Autodesk Inventor part; units mm, degrees
(part 3 of 6)
  spline S90 degree 5 poles (158.3441, 85.8402) (158.3513, 85.8419) (158.4053, 85.8546) (158.5062, 85.8783) (158.6539, 85.9125) (158.8488, 85.9569) (159.0837, 86.0091) (159.319, 86.0602) (159.5547, 86.1103) (159.7908, 86.1593) (160.0273, 86.2072) (160.2642, 86.2541) (160.5015, 86.3) (160.7391, 86.3449) (160.9771, 86.3887) (161.2155, 86.4315) (161.4542, 86.4734) (161.6932, 86.5143) (161.9326, 86.5542) (162.1723, 86.5932) (162.4124, 86.6312) (162.6527, 86.6682) (162.8934, 86.7044) (163.1343, 86.7396) (163.3756, 86.7739) (163.6172, 86.8073) (163.859, 86.8398) (164.1012, 86.8714) (164.3436, 86.9022) (164.5863, 86.932) (164.8293, 86.961) (165.0725, 86.9891) (165.3161, 87.0163) (165.5598, 87.0427) (165.8039, 87.0682) (166.0482, 87.0929) (166.2927, 87.1168) (166.5375, 87.1398) (166.7825, 87.162) (167.0278, 87.1834) (167.2733, 87.2039) (167.519, 87.2237) (167.765, 87.2426) (168.0604, 87.2644) (168.3069, 87.2815) (168.5042, 87.2946) (168.6523, 87.304) (168.7511, 87.3102) knots 0.383497 0.383497 0.383497 0.383497 0.383497 0.383497 0.385714 0.4 0.414286 0.428571 0.442857 0.457143 0.471429 0.485714 0.5 0.514286 0.528571 0.542857 0.557143 0.571429 0.585714 0.6 0.614286 0.628571 0.642857 0.657143 0.671429 0.685714 0.7 0.714286 0.728571 0.742857 0.757143 0.771429 0.785714 0.8 0.814286 0.828571 0.842857 0.857143 0.871429 0.885714 0.9 0.914286 0.928571 0.942857 0.957143 0.971429 1 1 1 1 1 1
  spline S91 degree 3 poles (156.5898, 86.6167) (156.7797, 86.2734) (157.3439, 85.8048) (158.0577, 85.7725) (158.3441, 85.8402) knots 0 0 0 0 0.571429 1 1 1 1
  arc A46 (156.5898, 86.6167) -> (155.8578, 87.927) centre (0, 0) ccw
  spline S92 degree 3 poles (156.1164, 89.828) (155.9086, 89.6196) (155.5618, 88.9948) (155.665, 88.2687) (155.8578, 87.927) knots 0 0 0 0 0.428571 1 1 1 1
  spline S93 degree 5 poles (156.1164, 89.828) (156.1216, 89.8333) (156.1608, 89.8726) (156.2338, 89.946) (156.3404, 90.0539) (156.4803, 90.1965) (156.648, 90.3692) (156.8149, 90.5427) (156.9811, 90.7172) (157.1466, 90.8926) (157.3115, 91.0689) (157.4756, 91.246) (157.6391, 91.424) (157.8019, 91.6028) (157.964, 91.7825) (158.1254, 91.963) (158.2862, 92.1443) (158.4464, 92.3264) (158.6059, 92.5094) (158.7647, 92.693) (158.923, 92.8775) (159.0805, 93.0627) (159.2375, 93.2487) (159.3938, 93.4354) (159.5495, 93.6229) (159.7046, 93.8111) (159.8591, 94) (160.013, 94.1896) (160.1663, 94.3799) (160.3189, 94.571) (160.471, 94.7627) (160.6225, 94.9551) (160.7733, 95.1482) (160.9236, 95.3419) (161.0733, 95.5363) (161.2224, 95.7314) (161.371, 95.9271) (161.5189, 96.1235) (161.6663, 96.3205) (161.8131, 96.5181) (161.9593, 96.7164) (162.1049, 96.9153) (162.25, 97.1148) (162.4234, 97.355) (162.5673, 97.5559) (162.6819, 97.7171) (162.7676, 97.8382) (162.8246, 97.9191) knots 0.383497 0.383497 0.383497 0.383497 0.383497 0.383497 0.385714 0.4 0.414286 0.428571 0.442857 0.457143 0.471429 0.485714 0.5 0.514286 0.528571 0.542857 0.557143 0.571429 0.585714 0.6 0.614286 0.628571 0.642857 0.657143 0.671429 0.685714 0.7 0.714286 0.728571 0.742857 0.757143 0.771429 0.785714 0.8 0.814286 0.828571 0.842857 0.857143 0.871429 0.885714 0.9 0.914286 0.928571 0.942857 0.957143 0.971429 1 1 1 1 1 1
  arc A47 (162.8246, 97.9191) -> (160.7388, 101.3067) centre (0, 0) ccw
  spline S94 degree 5 poles (150.4939, 98.9594) (150.501, 98.9618) (150.5537, 98.9791) (150.6522, 99.0112) (150.7965, 99.0578) (150.9869, 99.1185) (151.2165, 99.1905) (151.4466, 99.2614) (151.6772, 99.3313) (151.9084, 99.4001) (152.14, 99.4679) (152.372, 99.5348) (152.6045, 99.6006) (152.8375, 99.6654) (153.0709, 99.7293) (153.3048, 99.7922) (153.5391, 99.8541) (153.7738, 99.9152) (154.009, 99.9752) (154.2445, 100.0344) (154.4804, 100.0926) (154.7168, 100.1499) (154.9535, 100.2064) (155.1906, 100.2619) (155.4281, 100.3165) (155.666, 100.3703) (155.9042, 100.4232) (156.1428, 100.4752) (156.3817, 100.5264) (156.621, 100.5767) (156.8607, 100.6262) (157.1007, 100.6748) (157.341, 100.7226) (157.5817, 100.7696) (157.8227, 100.8157) (158.064, 100.861) (158.3056, 100.9056) (158.5476, 100.9492) (158.7898, 100.9921) (159.0324, 101.0342) (159.2753, 101.0755) (159.5184, 101.1161) (159.7619, 101.1558) (160.0544, 101.2025) (160.2985, 101.2405) (160.4941, 101.2703) (160.6409, 101.2922) (160.7388, 101.3067) knots 0.383497 0.383497 0.383497 0.383497 0.383497 0.383497 0.385714 0.4 0.414286 0.428571 0.442857 0.457143 0.471429 0.485714 0.5 0.514286 0.528571 0.542857 0.557143 0.571429 0.585714 0.6 0.614286 0.628571 0.642857 0.657143 0.671429 0.685714 0.7 0.714286 0.728571 0.742857 0.757143 0.771429 0.785714 0.8 0.814286 0.828571 0.842857 0.857143 0.871429 0.885714 0.9 0.914286 0.928571 0.942857 0.957143 0.971429 1 1 1 1 1 1
  spline S95 degree 3 poles (148.6801, 99.5844) (148.8984, 99.2584) (149.5003, 98.8394) (150.2143, 98.8677) (150.4939, 98.9594) knots 0 0 0 0 0.571429 1 1 1 1
  arc A48 (148.6801, 99.5844) -> (147.8396, 100.8279) centre (0, 0) ccw
  spline S96 degree 3 poles (147.936, 102.744) (147.7466, 102.5187) (147.4541, 101.8668) (147.6185, 101.1521) (147.8396, 100.8279) knots 0 0 0 0 0.428571 1 1 1 1
  spline S97 degree 5 poles (147.936, 102.744) (147.9408, 102.7497) (147.9765, 102.7921) (148.043, 102.8715) (148.1401, 102.988) (148.2674, 103.1421) (148.4198, 103.3283) (148.5714, 103.5154) (148.7222, 103.7033) (148.8723, 103.8921) (149.0216, 104.0817) (149.1701, 104.2721) (149.3179, 104.4634) (149.4649, 104.6554) (149.6112, 104.8481) (149.7568, 105.0417) (149.9016, 105.236) (150.0457, 105.431) (150.1892, 105.6268) (150.3319, 105.8233) (150.4739, 106.0205) (150.6152, 106.2184) (150.7558, 106.4171) (150.8957, 106.6164) (151.035, 106.8164) (151.1736, 107.017) (151.3115, 107.2184) (151.4487, 107.4203) (151.5853, 107.623) (151.7212, 107.8263) (151.8565, 108.0302) (151.9911, 108.2347) (152.125, 108.4399) (152.2583, 108.6457) (152.391, 108.8521) (152.523, 109.0591) (152.6544, 109.2668) (152.7852, 109.475) (152.9153, 109.6838) (153.0448, 109.8931) (153.1737, 110.1031) (153.302, 110.3136) (153.4296, 110.5247) (153.582, 110.7787) (153.7083, 110.9911) (153.8088, 111.1614) (153.8839, 111.2894) (153.9339, 111.3749) knots 0.383497 0.383497 0.383497 0.383497 0.383497 0.383497 0.385714 0.4 0.414286 0.428571 0.442857 0.457143 0.471429 0.485714 0.5 0.514286 0.528571 0.542857 0.557143 0.571429 0.585714 0.6 0.614286 0.628571 0.642857 0.657143 0.671429 0.685714 0.7 0.714286 0.728571 0.742857 0.757143 0.771429 0.785714 0.8 0.814286 0.828571 0.842857 0.857143 0.871429 0.885714 0.9 0.914286 0.928571 0.942857 0.957143 0.971429 1 1 1 1 1 1
  arc A49 (153.9339, 111.3749) -> (151.5683, 114.5734) centre (0, 0) ccw
  spline S98 degree 5 poles (141.5594, 111.3657) (141.5662, 111.3686) (141.6173, 111.3903) (141.7127, 111.4307) (141.8525, 111.4894) (142.0371, 111.566) (142.2598, 111.6572) (142.4831, 111.7474) (142.7069, 111.8366) (142.9314, 111.9248) (143.1564, 112.012) (143.382, 112.0982) (143.6081, 112.1835) (143.8347, 112.2679) (144.0619, 112.3513) (144.2896, 112.4339) (144.5178, 112.5154) (144.7465, 112.5961) (144.9756, 112.6759) (145.2053, 112.7549) (145.4355, 112.8329) (145.6661, 112.91) (145.8972, 112.9863) (146.1287, 113.0618) (146.3607, 113.1364) (146.5932, 113.2101) (146.8261, 113.283) (147.0594, 113.3551) (147.2931, 113.4263) (147.5273, 113.4968) (147.7619, 113.5664) (147.9969, 113.6352) (148.2323, 113.7032) (148.4681, 113.7704) (148.7043, 113.8368) (148.9409, 113.9025) (149.1779, 113.9673) (149.4153, 114.0314) (149.6531, 114.0946) (149.8912, 114.1572) (150.1297, 114.2189) (150.3685, 114.2799) (150.6078, 114.3401) (150.8953, 114.4115) (151.1353, 114.47) (151.3276, 114.5163) (151.472, 114.5506) (151.5683, 114.5734) knots 0.383497 0.383497 0.383497 0.383497 0.383497 0.383497 0.385714 0.4 0.414286 0.428571 0.442857 0.457143 0.471429 0.485714 0.5 0.514286 0.528571 0.542857 0.557143 0.571429 0.585714 0.6 0.614286 0.628571 0.642857 0.657143 0.671429 0.685714 0.7 0.714286 0.728571 0.742857 0.757143 0.771429 0.785714 0.8 0.814286 0.828571 0.842857 0.857143 0.871429 0.885714 0.9 0.914286 0.928571 0.942857 0.957143 0.971429 1 1 1 1 1 1
  spline S99 degree 3 poles (139.6991, 111.8346) (139.9443, 111.5283) (140.5796, 111.1618) (141.2886, 111.2506) (141.5594, 111.3657) knots 0 0 0 0 0.571429 1 1 1 1
  arc A50 (139.6991, 111.8346) -> (138.7562, 113.0023) centre (0, 0) ccw
  spline S100 degree 3 poles (138.6898, 114.9197) (138.5202, 114.6792) (138.284, 114.0048) (138.5084, 113.3066) (138.7562, 113.0023) knots 0 0 0 0 0.428571 1 1 1 1
  spline S101 degree 5 poles (138.6898, 114.9197) (138.6941, 114.9258) (138.726, 114.9711) (138.7856, 115.0558) (138.8724, 115.1802) (138.9862, 115.3445) (139.1223, 115.5429) (139.2575, 115.7422) (139.3918, 115.9423) (139.5253, 116.1431) (139.658, 116.3447) (139.7898, 116.547) (139.9209, 116.7501) (140.0511, 116.9538) (140.1805, 117.1583) (140.3091, 117.3635) (140.437, 117.5694) (140.564, 117.776) (140.6903, 117.9832) (140.8158, 118.1911) (140.9406, 118.3997) (141.0646, 118.6088) (141.1879, 118.8187) (141.3104, 119.0291) (141.4322, 119.2402) (141.5533, 119.4519) (141.6736, 119.6642) (141.7932, 119.8771) (141.9121, 120.0906) (142.0303, 120.3047) (142.1478, 120.5193) (142.2646, 120.7346) (142.3806, 120.9504) (142.496, 121.1667) (142.6107, 121.3836) (142.7247, 121.6011) (142.838, 121.8191) (142.9507, 122.0377) (143.0626, 122.2568) (143.1739, 122.4764) (143.2845, 122.6965) (143.3944, 122.9171) (143.5037, 123.1383) (143.6341, 123.4043) (143.7419, 123.6266) (143.8276, 123.8049) (143.8916, 123.9388) (143.9341, 124.0281) knots 0.383497 0.383497 0.383497 0.383497 0.383497 0.383497 0.385714 0.4 0.414286 0.428571 0.442857 0.457143 0.471429 0.485714 0.5 0.514286 0.528571 0.542857 0.557143 0.571429 0.585714 0.6 0.614286 0.628571 0.642857 0.657143 0.671429 0.685714 0.7 0.714286 0.728571 0.742857 0.757143 0.771429 0.785714 0.8 0.814286 0.828571 0.842857 0.857143 0.871429 0.885714 0.9 0.914286 0.928571 0.942857 0.957143 0.971429 1 1 1 1 1 1
  arc A51 (143.9341, 124.0281) -> (141.3058, 127.0145) centre (0, 0) ccw
  spline S102 degree 5 poles (131.6049, 122.9696) (131.6115, 122.9731) (131.6606, 122.999) (131.7522, 123.0473) (131.8865, 123.1177) (132.0639, 123.2097) (132.2781, 123.3194) (132.4929, 123.4282) (132.7084, 123.5361) (132.9246, 123.643) (133.1414, 123.749) (133.3588, 123.854) (133.5769, 123.9582) (133.7956, 124.0615) (134.0148, 124.1639) (134.2347, 124.2654) (134.4552, 124.3661) (134.6762, 124.4659) (134.8978, 124.5648) (135.1199, 124.6629) (135.3426, 124.7602) (135.5659, 124.8566) (135.7897, 124.9523) (136.014, 125.0471) (136.2388, 125.1411) (136.4642, 125.2342) (136.6901, 125.3266) (136.9164, 125.4182) (137.1433, 125.5091) (137.3706, 125.5991) (137.5985, 125.6884) (137.8268, 125.7768) (138.0556, 125.8646) (138.2849, 125.9515) (138.5146, 126.0377) (138.7448, 126.1232) (138.9754, 126.2079) (139.2065, 126.2919) (139.438, 126.3751) (139.67, 126.4576) (139.9024, 126.5393) (140.1352, 126.6203) (140.3685, 126.7006) (140.6489, 126.7961) (140.8831, 126.8748) (141.0708, 126.9372) (141.2117, 126.9837) (141.3058, 127.0145) knots 0.383497 0.383497 0.383497 0.383497 0.383497 0.383497 0.385714 0.4 0.414286 0.428571 0.442857 0.457143 0.471429 0.485714 0.5 0.514286 0.528571 0.542857 0.557143 0.571429 0.585714 0.6 0.614286 0.628571 0.642857 0.657143 0.671429 0.685714 0.7 0.714286 0.728571 0.742857 0.757143 0.771429 0.785714 0.8 0.814286 0.828571 0.842857 0.857143 0.871429 0.885714 0.9 0.914286 0.928571 0.942857 0.957143 0.971429 1 1 1 1 1 1
  spline S103 degree 3 poles (129.7116, 123.279) (129.9819, 122.9946) (130.646, 122.6833) (131.3448, 122.8319) (131.6049, 122.9696) knots 0 0 0 0 0.571429 1 1 1 1
  arc A52 (129.7116, 123.279) -> (128.6731, 124.3626) centre (0, 0) ccw
  spline S104 degree 3 poles (128.4443, 126.2674) (128.2957, 126.0134) (128.1176, 125.3214) (128.4004, 124.6447) (128.6731, 124.3626) knots 0 0 0 0 0.428571 1 1 1 1
  spline S105 degree 5 poles (128.4443, 126.2674) (128.448, 126.2738) (128.476, 126.3217) (128.5282, 126.4112) (128.6042, 126.5424) (128.7036, 126.7158) (128.8224, 126.9251) (128.9402, 127.1351) (129.0571, 127.3458) (129.173, 127.5573) (129.2881, 127.7694) (129.4024, 127.9821) (129.5157, 128.1956) (129.6282, 128.4097) (129.7398, 128.6244) (129.8505, 128.8398) (129.9605, 129.0558) (130.0695, 129.2724) (130.1778, 129.4895) (130.2852, 129.7073) (130.3919, 129.9257) (130.4977, 130.1447) (130.6027, 130.3642) (130.707, 130.5843) (130.8104, 130.8049) (130.9131, 131.0261) (131.015, 131.2479) (131.1161, 131.4702) (131.2165, 131.693) (131.3161, 131.9163) (131.415, 132.1401) (131.5131, 132.3645) (131.6104, 132.5894) (131.707, 132.8147) (131.8029, 133.0406) (131.898, 133.2669) (131.9925, 133.4938) (132.0862, 133.7211) (132.1791, 133.9489) (132.2714, 134.1771) (132.3629, 134.4059) (132.4538, 134.635) (132.5439, 134.8647) (132.6512, 135.1408) (132.7398, 135.3714) (132.81, 135.5563) (132.8624, 135.6951) (132.8972, 135.7878) knots 0.383497 0.383497 0.383497 0.383497 0.383497 0.383497 0.385714 0.4 0.414286 0.428571 0.442857 0.457143 0.471429 0.485714 0.5 0.514286 0.528571 0.542857 0.557143 0.571429 0.585714 0.6 0.614286 0.628571 0.642857 0.657143 0.671429 0.685714 0.7 0.714286 0.728571 0.742857 0.757143 0.771429 0.785714 0.8 0.814286 0.828571 0.842857 0.857143 0.871429 0.885714 0.9 0.914286 0.928571 0.942857 0.957143 0.971429 1 1 1 1 1 1
  arc A53 (132.8972, 135.7878) -> (130.0251, 138.5405) centre (0, 0) ccw
  spline S106 degree 5 poles (120.7023, 133.6875) (120.7086, 133.6915) (120.7552, 133.7215) (120.8424, 133.7774) (120.9703, 133.8589) (121.1393, 133.9656) (121.3433, 134.0931) (121.5482, 134.2197) (121.7538, 134.3455) (121.9601, 134.4703) (122.1671, 134.5943) (122.3748, 134.7175) (122.5833, 134.8398) (122.7924, 134.9612) (123.0022, 135.0818) (123.2127, 135.2016) (123.4238, 135.3206) (123.6356, 135.4388) (123.848, 135.5562) (124.061, 135.6728) (124.2747, 135.7886) (124.4889, 135.9036) (124.7038, 136.0179) (124.9193, 136.1314) (125.1353, 136.2441) (125.352, 136.3561) (125.5692, 136.4673) (125.787, 136.5777) (126.0053, 136.6875) (126.2242, 136.7965) (126.4437, 136.9047) (126.6637, 137.0123) (126.8842, 137.1191) (127.1053, 137.2252) (127.3268, 137.3305) (127.5489, 137.4352) (127.7716, 137.5392) (127.9947, 137.6424) (128.2183, 137.745) (128.4425, 137.8468) (128.6671, 137.948) (128.8922, 138.0485) (129.1178, 138.1483) (129.3891, 138.2672) (129.6158, 138.3655) (129.7975, 138.4435) (129.934, 138.5018) (130.0251, 138.5405) knots 0.383497 0.383497 0.383497 0.383497 0.383497 0.383497 0.385714 0.4 0.414286 0.428571 0.442857 0.457143 0.471429 0.485714 0.5 0.514286 0.528571 0.542857 0.557143 0.571429 0.585714 0.6 0.614286 0.628571 0.642857 0.657143 0.671429 0.685714 0.7 0.714286 0.728571 0.742857 0.757143 0.771429 0.785714 0.8 0.814286 0.828571 0.842857 0.857143 0.871429 0.885714 0.9 0.914286 0.928571 0.942857 0.957143 0.971429 1 1 1 1 1 1
  spline S107 degree 3 poles (118.7895, 133.8352) (119.083, 133.5748) (119.771, 133.3209) (120.4548, 133.5282) (120.7023, 133.6875) knots 0 0 0 0 0.571429 1 1 1 1
  arc A54 (118.7895, 133.8352) -> (117.6628, 134.8268) centre (0, 0) ccw
  spline S108 degree 3 poles (117.2733, 136.7053) (117.1468, 136.4396) (117.028, 135.7351) (117.3672, 135.0848) (117.6628, 134.8268) knots 0 0 0 0 0.428571 1 1 1 1
  spline S109 degree 5 poles (117.2733, 136.7053) (117.2765, 136.7121) (117.3004, 136.7622) (117.3447, 136.8558) (117.4093, 136.993) (117.4937, 137.1741) (117.5943, 137.3927) (117.6938, 137.612) (117.7924, 137.8319) (117.8901, 138.0524) (117.9868, 138.2735) (118.0825, 138.4952) (118.1774, 138.7175) (118.2713, 138.9403) (118.3643, 139.1637) (118.4564, 139.3877) (118.5476, 139.6122) (118.6379, 139.8373) (118.7274, 140.0629) (118.8159, 140.289) (118.9037, 140.5157) (118.9906, 140.7428) (119.0766, 140.9705) (119.1618, 141.1986) (119.2462, 141.4272) (119.3297, 141.6563) (119.4124, 141.8859) (119.4943, 142.116) (119.5754, 142.3465) (119.6558, 142.5774) (119.7353, 142.8089) (119.814, 143.0407) (119.8919, 143.2731) (119.9691, 143.5058) (120.0454, 143.739) (120.1211, 143.9726) (120.1959, 144.2066) (120.27, 144.441) (120.3433, 144.6759) (120.4159, 144.9112) (120.4877, 145.1468) (120.5587, 145.3829) (120.6291, 145.6193) (120.7126, 145.9035) (120.7813, 146.1409) (120.8356, 146.331) (120.876, 146.4738) (120.9029, 146.5691) knots 0.383497 0.383497 0.383497 0.383497 0.383497 0.383497 0.385714 0.4 0.414286 0.428571 0.442857 0.457143 0.471429 0.485714 0.5 0.514286 0.528571 0.542857 0.557143 0.571429 0.585714 0.6 0.614286 0.628571 0.642857 0.657143 0.671429 0.685714 0.7 0.714286 0.728571 0.742857 0.757143 0.771429 0.785714 0.8 0.814286 0.828571 0.842857 0.857143 0.871429 0.885714 0.9 0.914286 0.928571 0.942857 0.957143 0.971429 1 1 1 1 1 1
  arc A55 (120.9029, 146.5691) -> (117.8077, 149.0683) centre (0, 0) ccw
  spline S110 degree 5 poles (108.93, 143.4421) (108.9359, 143.4467) (108.9798, 143.4806) (109.062, 143.5436) (109.1825, 143.6357) (109.3418, 143.7563) (109.5343, 143.9007) (109.7277, 144.0442) (109.9219, 144.1869) (110.1168, 144.3288) (110.3126, 144.47) (110.5091, 144.6103) (110.7065, 144.7498) (110.9045, 144.8885) (111.1033, 145.0265) (111.3029, 145.1637) (111.5032, 145.3002) (111.7042, 145.4359) (111.9058, 145.5709) (112.1082, 145.7051) (112.3113, 145.8386) (112.515, 145.9714) (112.7194, 146.1035) (112.9245, 146.2348) (113.1302, 146.3655) (113.3366, 146.4954) (113.5436, 146.6247) (113.7512, 146.7532) (113.9595, 146.8811) (114.1683, 147.0082) (114.3778, 147.1347) (114.5879, 147.2605) (114.7986, 147.3856) (115.0098, 147.5101) (115.2217, 147.6339) (115.4341, 147.757) (115.6471, 147.8795) (115.8607, 148.0013) (116.0748, 148.1224) (116.2895, 148.2429) (116.5048, 148.3628) (116.7206, 148.482) (116.9369, 148.6006) (117.1971, 148.7421) (117.4146, 148.8592) (117.5891, 148.9524) (117.7202, 149.022) (117.8077, 149.0683) knots 0.383497 0.383497 0.383497 0.383497 0.383497 0.383497 0.385714 0.4 0.414286 0.428571 0.442857 0.457143 0.471429 0.485714 0.5 0.514286 0.528571 0.542857 0.557143 0.571429 0.585714 0.6 0.614286 0.628571 0.642857 0.657143 0.671429 0.685714 0.7 0.714286 0.728571 0.742857 0.757143 0.771429 0.785714 0.8 0.814286 0.828571 0.842857 0.857143 0.871429 0.885714 0.9 0.914286 0.928571 0.942857 0.957143 0.971429 1 1 1 1 1 1
  spline S111 degree 3 poles (107.0115, 143.4271) (107.326, 143.1925) (108.0331, 142.9979) (108.6969, 143.2625) (108.93, 143.4421) knots 0 0 0 0 0.571429 1 1 1 1
  arc A56 (107.0115, 143.4271) -> (105.8048, 144.3196) centre (0, 0) ccw
  spline S112 degree 3 poles (105.2574, 146.1583) (105.1539, 145.8829) (105.0953, 145.1707) (105.4884, 144.5516) (105.8048, 144.3196) knots 0 0 0 0 0.428571 1 1 1 1
  spline S113 degree 5 poles (105.2574, 146.1583) (105.26, 146.1653) (105.2796, 146.2173) (105.3158, 146.3143) (105.3685, 146.4565) (105.4373, 146.6441) (105.5189, 146.8705) (105.5995, 147.0974) (105.6791, 147.3248) (105.7577, 147.5528) (105.8353, 147.7813) (105.9119, 148.0103) (105.9876, 148.2399) (106.0622, 148.4699) (106.1359, 148.7004) (106.2087, 148.9314) (106.2806, 149.1628) (106.3515, 149.3947) (106.4215, 149.6271) (106.4906, 149.8599) (106.5588, 150.0932) (106.6261, 150.3269) (106.6925, 150.561) (106.758, 150.7955) (106.8227, 151.0305) (106.8865, 151.2659) (106.9495, 151.5016) (107.0116, 151.7378) (107.0728, 151.9744) (107.1333, 152.2113) (107.1929, 152.4487) (107.2516, 152.6864) (107.3096, 152.9245) (107.3667, 153.1629) (107.4231, 153.4017) (107.4786, 153.6409) (107.5333, 153.8804) (107.5872, 154.1203) (107.6404, 154.3605) (107.6927, 154.6011) (107.7443, 154.842) (107.7951, 155.0832) (107.8451, 155.3248) (107.9042, 155.6151) (107.9525, 155.8573) (107.9906, 156.0514) (108.0187, 156.1971) (108.0374, 156.2944) knots 0.383497 0.383497 0.383497 0.383497 0.383497 0.383497 0.385714 0.4 0.414286 0.428571 0.442857 0.457143 0.471429 0.485714 0.5 0.514286 0.528571 0.542857 0.557143 0.571429 0.585714 0.6 0.614286 0.628571 0.642857 0.657143 0.671429 0.685714 0.7 0.714286 0.728571 0.742857 0.757143 0.771429 0.785714 0.8 0.814286 0.828571 0.842857 0.857143 0.871429 0.885714 0.9 0.914286 0.928571 0.942857 0.957143 0.971429 1 1 1 1 1 1
  arc A57 (108.0374, 156.2944) -> (104.7414, 158.5221) centre (0, 0) ccw
  spline S114 degree 5 poles (96.3728, 152.1633) (96.3783, 152.1683) (96.4192, 152.2058) (96.4957, 152.2756) (96.608, 152.3776) (96.7565, 152.5113) (96.9361, 152.6715) (97.1166, 152.8309) (97.298, 152.9895) (97.4802, 153.1475) (97.6633, 153.3047) (97.8472, 153.4611) (98.032, 153.6169) (98.2176, 153.7719) (98.404, 153.9263) (98.5912, 154.0799) (98.7792, 154.2329) (98.9679, 154.3852) (99.1574, 154.5368) (99.3477, 154.6877) (99.5387, 154.8379) (99.7304, 154.9875) (99.9229, 155.1364) (100.1161, 155.2847) (100.31, 155.4323) (100.5046, 155.5793) (100.6999, 155.7256) (100.8959, 155.8713) (101.0926, 156.0164) (101.2899, 156.1608) (101.4879, 156.3046) (101.6865, 156.4477) (101.8858, 156.5903) (102.0858, 156.7322) (102.2864, 156.8735) (102.4876, 157.0142) (102.6895, 157.1543) (102.8919, 157.2938) (103.095, 157.4326) (103.2987, 157.5709) (103.503, 157.7086) (103.7079, 157.8457) (103.9134, 157.9822) (104.1607, 158.1452) (104.3675, 158.2804) (104.5334, 158.388) (104.6581, 158.4685) (104.7414, 158.5221) knots 0.383497 0.383497 0.383497 0.383497 0.383497 0.383497 0.385714 0.4 0.414286 0.428571 0.442857 0.457143 0.471429 0.485714 0.5 0.514286 0.528571 0.542857 0.557143 0.571429 0.585714 0.6 0.614286 0.628571 0.642857 0.657143 0.671429 0.685714 0.7 0.714286 0.728571 0.742857 0.757143 0.771429 0.785714 0.8 0.814286 0.828571 0.842857 0.857143 0.871429 0.885714 0.9 0.914286 0.928571 0.942857 0.957143 0.971429 1 1 1 1 1 1
  spline S115 degree 3 poles (94.4626, 151.9857) (94.7958, 151.7785) (95.5169, 151.6446) (96.1558, 151.9645) (96.3728, 152.1633) knots 0 0 0 0 0.571429 1 1 1 1
  arc A58 (94.4626, 151.9857) -> (93.1845, 152.7726) centre (0, 0) ccw
  spline S116 degree 3 poles (92.4831, 154.5582) (92.4034, 154.275) (92.4054, 153.5605) (92.8495, 152.9769) (93.1845, 152.7726) knots 0 0 0 0 0.428571 1 1 1 1
  spline S117 degree 5 poles (92.4831, 154.5582) (92.4852, 154.5654) (92.5002, 154.6188) (92.5281, 154.7186) (92.5686, 154.8647) (92.6211, 155.0575) (92.6833, 155.29) (92.7444, 155.5229) (92.8044, 155.7563) (92.8634, 155.9901) (92.9213, 156.2244) (92.9782, 156.4591) (93.0341, 156.6942) (93.089, 156.9297) (93.1429, 157.1657) (93.1958, 157.402) (93.2478, 157.6387) (93.2988, 157.8758) (93.3488, 158.1133) (93.3979, 158.3511) (93.4461, 158.5893) (93.4933, 158.8279) (93.5397, 159.0668) (93.5851, 159.306) (93.6296, 159.5456) (93.6732, 159.7855) (93.716, 160.0258) (93.7578, 160.2664) (93.7988, 160.5073) (93.8389, 160.7485) (93.8782, 160.9901) (93.9166, 161.2319) (93.9541, 161.474) (93.9908, 161.7165) (94.0267, 161.9592) (94.0617, 162.2022) (94.096, 162.4455) (94.1293, 162.6891) (94.1619, 162.933) (94.1937, 163.1771) (94.2246, 163.4215) (94.2548, 163.6662) (94.2842, 163.9111) (94.3184, 164.2054) (94.346, 164.4509) (94.3674, 164.6475) (94.3832, 164.7951) (94.3935, 164.8935) knots 0.383497 0.383497 0.383497 0.383497 0.383497 0.383497 0.385714 0.4 0.414286 0.428571 0.442857 0.457143 0.471429 0.485714 0.5 0.514286 0.528571 0.542857 0.557143 0.571429 0.585714 0.6 0.614286 0.628571 0.642857 0.657143 0.671429 0.685714 0.7 0.714286 0.728571 0.742857 0.757143 0.771429 0.785714 0.8 0.814286 0.828571 0.842857 0.857143 0.871429 0.885714 0.9 0.914286 0.928571 0.942857 0.957143 0.971429 1 1 1 1 1 1
  arc A59 (94.3935, 164.8935) -> (90.9204, 166.8337) centre (0, 0) ccw
  spline S118 degree 5 poles (83.1213, 159.7881) (83.1263, 159.7936) (83.1639, 159.8344) (83.2342, 159.9104) (83.3374, 160.0215) (83.4741, 160.1674) (83.6394, 160.3422) (83.8058, 160.5163) (83.973, 160.6898) (84.1412, 160.8626) (84.3103, 161.0348) (84.4803, 161.2063) (84.6512, 161.3772) (84.823, 161.5474) (84.9956, 161.717) (85.1691, 161.886) (85.3434, 162.0543) (85.5186, 162.2221) (85.6946, 162.3892) (85.8714, 162.5557) (86.0489, 162.7216) (86.2273, 162.8869) (86.4065, 163.0516) (86.5864, 163.2157) (86.7671, 163.3793) (86.9485, 163.5422) (87.1307, 163.7046) (87.3136, 163.8663) (87.4973, 164.0275) (87.6816, 164.1882) (87.8667, 164.3482) (88.0525, 164.5077) (88.239, 164.6667) (88.4262, 164.825) (88.6141, 164.9829) (88.8027, 165.1401) (88.9919, 165.2968) (89.1818, 165.453) (89.3724, 165.6086) (89.5636, 165.7636) (89.7555, 165.9181) (89.9481, 166.0721) (90.1412, 166.2255) (90.3738, 166.409) (90.5684, 166.5612) (90.7246, 166.6825) (90.842, 166.7733) (90.9204, 166.8337) knots 0.383497 0.383497 0.383497 0.383497 0.383497 0.383497 0.385714 0.4 0.414286 0.428571 0.442857 0.457143 0.471429 0.485714 0.5 0.514286 0.528571 0.542857 0.557143 0.571429 0.585714 0.6 0.614286 0.628571 0.642857 0.657143 0.671429 0.685714 0.7 0.714286 0.728571 0.742857 0.757143 0.771429 0.785714 0.8 0.814286 0.828571 0.842857 0.857143 0.871429 0.885714 0.9 0.914286 0.928571 0.942857 0.957143 0.971429 1 1 1 1 1 1
  spline S119 degree 3 poles (81.233, 159.4491) (81.5826, 159.271) (82.3124, 159.1987) (82.9219, 159.5716) (83.1213, 159.7881) knots 0 0 0 0 0.571429 1 1 1 1
  arc A60 (81.233, 159.4491) -> (79.8928, 160.1248) centre (0, 0) ccw
  spline S120 degree 3 poles (79.0425, 161.8446) (78.987, 161.5556) (79.0496, 160.8438) (79.5417, 160.3) (79.8928, 160.1248) knots 0 0 0 0 0.428571 1 1 1 1
  spline S121 degree 5 poles (79.0425, 161.8446) (79.0439, 161.8519) (79.0544, 161.9064) (79.0737, 162.0081) (79.1016, 162.1572) (79.1377, 162.3537) (79.1799, 162.5907) (79.221, 162.8279) (79.261, 163.0656) (79.2999, 163.3036) (79.3378, 163.5419) (79.3746, 163.7806) (79.4104, 164.0196) (79.4451, 164.2589) (79.4788, 164.4985) (79.5115, 164.7385) (79.5432, 164.9788) (79.5739, 165.2193) (79.6036, 165.4602) (79.6323, 165.7013) (79.6601, 165.9428) (79.687, 166.1845) (79.7129, 166.4264) (79.7378, 166.6687) (79.7619, 166.9112) (79.785, 167.154) (79.8072, 167.397) (79.8285, 167.6402) (79.8489, 167.8838) (79.8684, 168.1275) (79.8871, 168.3715) (79.9048, 168.6157) (79.9217, 168.8602) (79.9377, 169.1049) (79.9529, 169.3498) (79.9672, 169.5949) (79.9806, 169.8402) (79.9932, 170.0858) (80.005, 170.3315) (80.016, 170.5775) (80.0261, 170.8236) (80.0354, 171.07) (80.0439, 171.3165) (80.0531, 171.6126) (80.0597, 171.8595) (80.0644, 172.0573) (80.0675, 172.2057) (80.0695, 172.3046) knots 0.383497 0.383497 0.383497 0.383497 0.383497 0.383497 0.385714 0.4 0.414286 0.428571 0.442857 0.457143 0.471429 0.485714 0.5 0.514286 0.528571 0.542857 0.557143 0.571429 0.585714 0.6 0.614286 0.628571 0.642857 0.657143 0.671429 0.685714 0.7 0.714286 0.728571 0.742857 0.757143 0.771429 0.785714 0.8 0.814286 0.828571 0.842857 0.857143 0.871429 0.885714 0.9 0.914286 0.928571 0.942857 0.957143 0.971429 1 1 1 1 1 1
  arc A61 (80.0695, 172.3046) -> (76.4444, 173.9432) centre (0, 0) ccw
  spline S122 degree 5 poles (69.2708, 166.2616) (69.2754, 166.2675) (69.3094, 166.3114) (69.373, 166.3931) (69.4664, 166.5126) (69.5902, 166.6695) (69.7401, 166.8577) (69.8911, 167.0453) (70.0431, 167.2323) (70.196, 167.4188) (70.3499, 167.6047) (70.5047, 167.79) (70.6605, 167.9747) (70.8172, 168.1589) (70.9749, 168.3426) (71.1334, 168.5256) (71.2928, 168.7082) (71.4531, 168.8901) (71.6143, 169.0716) (71.7763, 169.2525) (71.9392, 169.4328) (72.1029, 169.6127) (72.2674, 169.792) (72.4328, 169.9708) (72.599, 170.149) (72.7659, 170.3268) (72.9337, 170.504) (73.1022, 170.6807) (73.2715, 170.8569) (73.4416, 171.0326) (73.6125, 171.2078) (73.7841, 171.3825) (73.9564, 171.5567) (74.1295, 171.7303) (74.3033, 171.9035) (74.4779, 172.0762) (74.6532, 172.2484) (74.8292, 172.4201) (75.0059, 172.5913) (75.1833, 172.762) (75.3613, 172.9322) (75.5401, 173.1019) (75.7196, 173.2712) (75.9358, 173.4737) (76.1168, 173.6419) (76.2621, 173.776) (76.3714, 173.8764) (76.4444, 173.9432) knots 0.383497 0.383497 0.383497 0.383497 0.383497 0.383497 0.385714 0.4 0.414286 0.428571 0.442857 0.457143 0.471429 0.485714 0.5 0.514286 0.528571 0.542857 0.557143 0.571429 0.585714 0.6 0.614286 0.628571 0.642857 0.657143 0.671429 0.685714 0.7 0.714286 0.728571 0.742857 0.757143 0.771429 0.785714 0.8 0.814286 0.828571 0.842857 0.857143 0.871429 0.885714 0.9 0.914286 0.928571 0.942857 0.957143 0.971429 1 1 1 1 1 1
  spline S123 degree 3 poles (67.4181, 165.7637) (67.7816, 165.6159) (68.5149, 165.6058) (69.0905, 166.0291) (69.2708, 166.2616) knots 0 0 0 0 0.571429 1 1 1 1
  arc A62 (67.4181, 165.7637) -> (66.0255, 166.3233) centre (0, 0) ccw
  spline S124 degree 3 poles (65.0324, 167.9648) (65.0016, 167.6721) (65.1243, 166.9682) (65.6608, 166.4681) (66.0255, 166.3233) knots 0 0 0 0 0.428571 1 1 1 1
  spline S125 degree 5 poles (65.0324, 167.9648) (65.0332, 167.9722) (65.039, 168.0274) (65.0496, 168.1304) (65.0648, 168.2813) (65.084, 168.4802) (65.106, 168.7198) (65.1268, 168.9598) (65.1466, 169.1999) (65.1652, 169.4404) (65.1827, 169.681) (65.1991, 169.922) (65.2145, 170.1631) (65.2288, 170.4046) (65.242, 170.6462) (65.2542, 170.8881) (65.2654, 171.1302) (65.2756, 171.3725) (65.2848, 171.615) (65.293, 171.8577) (65.3002, 172.1006) (65.3065, 172.3437) (65.3118, 172.587) (65.3161, 172.8305) (65.3195, 173.0742) (65.3219, 173.318) (65.3234, 173.5621) (65.324, 173.8063) (65.3237, 174.0506) (65.3225, 174.2952) (65.3204, 174.5398) (65.3173, 174.7847) (65.3134, 175.0297) (65.3086, 175.2749) (65.303, 175.5202) (65.2964, 175.7656) (65.289, 176.0112) (65.2808, 176.2569) (65.2717, 176.5028) (65.2617, 176.7488) (65.2509, 176.9949) (65.2393, 177.2411) (65.2268, 177.4875) (65.2109, 177.7833) (65.1966, 178.03) (65.1845, 178.2274) (65.175, 178.3755) (65.1686, 178.4742) knots 0.383497 0.383497 0.383497 0.383497 0.383497 0.383497 0.385714 0.4 0.414286 0.428571 0.442857 0.457143 0.471429 0.485714 0.5 0.514286 0.528571 0.542857 0.557143 0.571429 0.585714 0.6 0.614286 0.628571 0.642857 0.657143 0.671429 0.685714 0.7 0.714286 0.728571 0.742857 0.757143 0.771429 0.785714 0.8 0.814286 0.828571 0.842857 0.857143 0.871429 0.885714 0.9 0.914286 0.928571 0.942857 0.957143 0.971429 1 1 1 1 1 1
  arc A63 (65.1686, 178.4742) -> (61.4176, 179.7995) centre (0, 0) ccw
  spline S126 degree 5 poles (54.9213, 171.5373) (54.9254, 171.5435) (54.9555, 171.5901) (55.012, 171.6769) (55.0949, 171.8039) (55.2049, 171.9707) (55.3384, 172.171) (55.4729, 172.3707) (55.6084, 172.57) (55.745, 172.7687) (55.8826, 172.967) (56.0211, 173.1648) (56.1607, 173.362) (56.3012, 173.5589) (56.4427, 173.7552) (56.5852, 173.951) (56.7285, 174.1464) (56.8728, 174.3414) (57.018, 174.5358) (57.1641, 174.7298) (57.3111, 174.9233) (57.459, 175.1164) (57.6077, 175.309) (57.7573, 175.5012) (57.9078, 175.6929) (58.0591, 175.8842) (58.2112, 176.075) (58.3641, 176.2653) (58.5179, 176.4553) (58.6725, 176.6448) (58.8278, 176.8338) (58.984, 177.0224) (59.141, 177.2106) (59.2987, 177.3983) (59.4572, 177.5856) (59.6165, 177.7724) (59.7765, 177.9589) (59.9373, 178.1449) (60.0989, 178.3304) (60.2612, 178.5156) (60.4242, 178.7003) (60.5879, 178.8846) (60.7524, 179.0684) (60.9506, 179.2886) (61.1167, 179.4715) (61.2501, 179.6175) (61.3505, 179.7268) (61.4176, 179.7995) knots 0.383497 0.383497 0.383497 0.383497 0.383497 0.383497 0.385714 0.4 0.414286 0.428571 0.442857 0.457143 0.471429 0.485714 0.5 0.514286 0.528571 0.542857 0.557143 0.571429 0.585714 0.6 0.614286 0.628571 0.642857 0.657143 0.671429 0.685714 0.7 0.714286 0.728571 0.742857 0.757143 0.771429 0.785714 0.8 0.814286 0.828571 0.842857 0.857143 0.871429 0.885714 0.9 0.914286 0.928571 0.942857 0.957143 0.971429 1 1 1 1 1 1
  spline S127 degree 3 poles (53.1175, 170.884) (53.4922, 170.7676) (54.2237, 170.8197) (54.7614, 171.2902) (54.9213, 171.5373) knots 0 0 0 0 0.571429 1 1 1 1
  arc A64 (53.1175, 170.884) -> (51.6824, 171.3235) centre (0, 0) ccw
  spline S128 degree 3 poles (50.5537, 172.8748) (50.5479, 172.5806) (50.7298, 171.8896) (51.3067, 171.4368) (51.6824, 171.3235) knots 0 0 0 0 0.428571 1 1 1 1
  spline S129 degree 5 poles (50.5537, 172.8748) (50.5538, 172.8823) (50.5549, 172.9378) (50.5568, 173.0413) (50.5591, 173.1929) (50.5614, 173.3928) (50.563, 173.6334) (50.5634, 173.8742) (50.5627, 174.1152) (50.5609, 174.3563) (50.5579, 174.5976) (50.5538, 174.8391) (50.5487, 175.0807) (50.5425, 175.3225) (50.5352, 175.5644) (50.5268, 175.8064) (50.5175, 176.0486) (50.5071, 176.2908) (50.4957, 176.5333) (50.4832, 176.7758) (50.4698, 177.0184) (50.4554, 177.2612) (50.4401, 177.5041) (50.4237, 177.7471) (50.4064, 177.9901) (50.3882, 178.2333) (50.369, 178.4766) (50.3489, 178.72) (50.3279, 178.9634) (50.3059, 179.207) (50.283, 179.4506) (50.2593, 179.6943) (50.2346, 179.9381) (50.209, 180.182) (50.1826, 180.4259) (50.1552, 180.6699) (50.127, 180.914) (50.098, 181.1581) (50.0681, 181.4024) (50.0373, 181.6466) (50.0056, 181.8909) (49.9732, 182.1353) (49.9399, 182.3797) (49.8989, 182.6731) (49.8637, 182.9177) (49.8349, 183.1133) (49.813, 183.2601) (49.7981, 183.358) knots 0.383497 0.383497 0.383497 0.383497 0.383497 0.383497 0.385714 0.4 0.414286 0.428571 0.442857 0.457143 0.471429 0.485714 0.5 0.514286 0.528571 0.542857 0.557143 0.571429 0.585714 0.6 0.614286 0.628571 0.642857 0.657143 0.671429 0.685714 0.7 0.714286 0.728571 0.742857 0.757143 0.771429 0.785714 0.8 0.814286 0.828571 0.842857 0.857143 0.871429 0.885714 0.9 0.914286 0.928571 0.942857 0.957143 0.971429 1 1 1 1 1 1
  arc A65 (49.7981, 183.358) -> (45.9483, 184.3604) centre (0, 0) ccw
  spline S130 degree 5 poles (40.1761, 175.577) (40.1796, 175.5835) (40.2057, 175.6325) (40.2546, 175.7238) (40.3265, 175.8573) (40.4219, 176.0329) (40.5379, 176.2437) (40.655, 176.4542) (40.7731, 176.6642) (40.8924, 176.8738) (41.0126, 177.083) (41.1339, 177.2918) (41.2563, 177.5003) (41.3796, 177.7083) (41.5039, 177.9159) (41.6292, 178.1231) (41.7555, 178.33) (41.8828, 178.5364) (42.011, 178.7425) (42.1401, 178.9482) (42.2701, 179.1535) (42.4011, 179.3584) (42.5329, 179.5629) (42.6657, 179.7671) (42.7994, 179.9709) (42.9339, 180.1743) (43.0693, 180.3773) (43.2055, 180.58) (43.3426, 180.7823) (43.4806, 180.9842) (43.6194, 181.1857) (43.759, 181.3869) (43.8994, 181.5877) (44.0407, 181.7881) (44.1827, 181.9882) (44.3256, 182.1879) (44.4692, 182.3872) (44.6137, 182.5861) (44.7589, 182.7847) (44.9049, 182.983) (45.0517, 183.1809) (45.1992, 183.3784) (45.3475, 183.5755) (45.5263, 183.8117) (45.6763, 184.008) (45.7969, 184.1648) (45.8876, 184.2822) (45.9483, 184.3604) knots 0.383497 0.383497 0.383497 0.383497 0.383497 0.383497 0.385714 0.4 0.414286 0.428571 0.442857 0.457143 0.471429 0.485714 0.5 0.514286 0.528571 0.542857 0.557143 0.571429 0.585714 0.6 0.614286 0.628571 0.642857 0.657143 0.671429 0.685714 0.7 0.714286 0.728571 0.742857 0.757143 0.771429 0.785714 0.8 0.814286 0.828571 0.842857 0.857143 0.871429 0.885714 0.9 0.914286 0.928571 0.942857 0.957143 0.971429 1 1 1 1 1 1
  spline S131 degree 3 poles (38.4341, 174.7731) (38.8174, 174.6888) (39.5419, 174.8028) (40.0377, 175.3172) (40.1761, 175.577) knots 0 0 0 0 0.571429 1 1 1 1
  arc A66 (38.4341, 174.7731) -> (36.967, 175.0893) centre (0, 0) ccw
  spline S132 degree 3 poles (35.7108, 176.5393) (35.7299, 176.2456) (35.9698, 175.5726) (36.583, 175.1703) (36.967, 175.0893) knots 0 0 0 0 0.428571 1 1 1 1
  spline S133 degree 5 poles (35.7108, 176.5393) (35.7103, 176.5467) (35.7067, 176.6021) (35.6998, 176.7054) (35.6892, 176.8567) (35.6746, 177.056) (35.6557, 177.2959) (35.6357, 177.5359) (35.6146, 177.776) (35.5923, 178.0161) (35.5688, 178.2563) (35.5443, 178.4965) (35.5187, 178.7368) (35.492, 178.9772) (35.4642, 179.2176) (35.4354, 179.458) (35.4055, 179.6985) (35.3746, 179.9391) (35.3427, 180.1796) (35.3097, 180.4202) (35.2758, 180.6609) (35.2409, 180.9015) (35.205, 181.1422) (35.1681, 181.383) (35.1302, 181.6237) (35.0914, 181.8645) (35.0517, 182.1052) (35.011, 182.346) (34.9694, 182.5868) (34.9269, 182.8276) (34.8834, 183.0684) (34.8391, 183.3093) (34.7938, 183.5501) (34.7476, 183.7909) (34.7006, 184.0317) (34.6527, 184.2725) (34.6039, 184.5133) (34.5542, 184.7541) (34.5037, 184.9949) (34.4523, 185.2357) (34.4001, 185.4764) (34.347, 185.7172) (34.2931, 185.9579) (34.2274, 186.2468) (34.1716, 186.4874) (34.1263, 186.68) (34.092, 186.8243) (34.0689, 186.9206) knots 0.383497 0.383497 0.383497 0.383497 0.383497 0.383497 0.385714 0.4 0.414286 0.428571 0.442857 0.457143 0.471429 0.485714 0.5 0.514286 0.528571 0.542857 0.557143 0.571429 0.585714 0.6 0.614286 0.628571 0.642857 0.657143 0.671429 0.685714 0.7 0.714286 0.728571 0.742857 0.757143 0.771429 0.785714 0.8 0.814286 0.828571 0.842857 0.857143 0.871429 0.885714 0.9 0.914286 0.928571 0.942857 0.957143 0.971429 1 1 1 1 1 1
  arc A67 (34.0689, 186.9206) -> (30.1479, 187.5929) centre (0, 0) ccw
  spline S134 degree 5 poles (25.1414, 178.3516) (25.1443, 178.3585) (25.1662, 178.4095) (25.2071, 178.5046) (25.2675, 178.6437) (25.3477, 178.8267) (25.4454, 179.0467) (25.5442, 179.2663) (25.6441, 179.4856) (25.7451, 179.7045) (25.8472, 179.9232) (25.9503, 180.1416) (26.0546, 180.3596) (26.1598, 180.5773) (26.2661, 180.7947) (26.3734, 181.0119) (26.4817, 181.2287) (26.5909, 181.4452) (26.7012, 181.6614) (26.8124, 181.8773) (26.9246, 182.0928) (27.0377, 182.3081) (27.1517, 182.5231) (27.2667, 182.7378) (27.3826, 182.9522) (27.4994, 183.1663) (27.617, 183.38) (27.7356, 183.5935) (27.8551, 183.8067) (27.9754, 184.0196) (28.0966, 184.2322) (28.2187, 184.4444) (28.3416, 184.6564) (28.4653, 184.8681) (28.5899, 185.0795) (28.7153, 185.2906) (28.8415, 185.5014) (28.9686, 185.7119) (29.0964, 185.9221) (29.2251, 186.132) (29.3545, 186.3416) (29.4848, 186.5509) (29.6158, 186.7599) (29.774, 187.0104) (29.9068, 187.2187) (30.0136, 187.3852) (30.0941, 187.5098) (30.1479, 187.5929) knots 0.383497 0.383497 0.383497 0.383497 0.383497 0.383497 0.385714 0.4 0.414286 0.428571 0.442857 0.457143 0.471429 0.485714 0.5 0.514286 0.528571 0.542857 0.557143 0.571429 0.585714 0.6 0.614286 0.628571 0.642857 0.657143 0.671429 0.685714 0.7 0.714286 0.728571 0.742857 0.757143 0.771429 0.785714 0.8 0.814286 0.828571 0.842857 0.857143 0.871429 0.885714 0.9 0.914286 0.928571 0.942857 0.957143 0.971429 1 1 1 1 1 1
  spline S135 degree 3 poles (23.4739, 177.4029) (23.8629, 177.3514) (24.5751, 177.5264) (25.0255, 178.0811) (25.1414, 178.3516) knots 0 0 0 0 0.571429 1 1 1 1
  arc A68 (23.4739, 177.4029) -> (21.9852, 177.5935) centre (0, 0) ccw
  spline S136 degree 3 poles (20.6105, 178.9318) (20.6545, 178.6408) (20.9506, 177.9906) (21.5958, 177.6418) (21.9852, 177.5935) knots 0 0 0 0 0.428571 1 1 1 1
  spline S137 degree 5 poles (20.6105, 178.9318) (20.6094, 178.9392) (20.6011, 178.994) (20.5855, 179.0964) (20.5622, 179.2463) (20.5306, 179.4436) (20.4915, 179.681) (20.4512, 179.9185) (20.4098, 180.1558) (20.3672, 180.3932) (20.3235, 180.6305) (20.2787, 180.8678) (20.2328, 181.1051) (20.1858, 181.3423) (20.1378, 181.5795) (20.0886, 181.8167) (20.0385, 182.0537) (19.9873, 182.2908) (19.9351, 182.5278) (19.8818, 182.7647) (19.8276, 183.0016) (19.7724, 183.2385) (19.7162, 183.4753) (19.659, 183.712) (19.6009, 183.9487) (19.5418, 184.1853) (19.4818, 184.4218) (19.4209, 184.6583) (19.359, 184.8947) (19.2962, 185.131) (19.2325, 185.3673) (19.1678, 185.6034) (19.1023, 185.8396) (19.0359, 186.0756) (18.9686, 186.3116) (18.9004, 186.5474) (18.8314, 186.7832) (18.7615, 187.019) (18.6907, 187.2546) (18.6191, 187.4901) (18.5466, 187.7256) (18.4733, 187.961) (18.3992, 188.1963) (18.3092, 188.4785) (18.2332, 188.7136) (18.1718, 188.9016) (18.1253, 189.0425) (18.0942, 189.1365) knots 0.383497 0.383497 0.383497 0.383497 0.383497 0.383497 0.385714 0.4 0.414286 0.428571 0.442857 0.457143 0.471429 0.485714 0.5 0.514286 0.528571 0.542857 0.557143 0.571429 0.585714 0.6 0.614286 0.628571 0.642857 0.657143 0.671429 0.685714 0.7 0.714286 0.728571 0.742857 0.757143 0.771429 0.785714 0.8 0.814286 0.828571 0.842857 0.857143 0.871429 0.885714 0.9 0.914286 0.928571 0.942857 0.957143 0.971429 1 1 1 1 1 1
  arc A69 (18.0942, 189.1365) -> (14.1303, 189.4738) centre (0, 0) ccw
  spline S138 degree 5 poles (9.9255, 179.8412) (9.9279, 179.8483) (9.9453, 179.901) (9.9781, 179.9992) (10.0264, 180.143) (10.0908, 180.3322) (10.1695, 180.5596) (10.2493, 180.7868) (10.3303, 181.0137) (10.4123, 181.2405) (10.4955, 181.467) (10.5798, 181.6933) (10.6651, 181.9194) (10.7515, 182.1453) (10.839, 182.3709) (10.9275, 182.5964) (11.017, 182.8216) (11.1075, 183.0466) (11.199, 183.2713) (11.2915, 183.4959) (11.385, 183.7202) (11.4795, 183.9443) (11.5749, 184.1682) (11.6712, 184.3919) (11.7685, 184.6153) (11.8667, 184.8385) (11.9658, 185.0615) (12.0659, 185.2843) (12.1668, 185.5068) (12.2687, 185.7291) (12.3714, 185.9512) (12.475, 186.1731) (12.5795, 186.3947) (12.6848, 186.6161) (12.791, 186.8373) (12.8981, 187.0583) (13.006, 187.279) (13.1147, 187.4996) (13.2243, 187.7198) (13.3347, 187.9399) (13.4459, 188.1597) (13.5579, 188.3793) (13.6708, 188.5987) (13.8071, 188.8617) (13.9218, 189.0805) (14.0141, 189.2554) (14.0837, 189.3865) (14.1303, 189.4738) knots 0.383497 0.383497 0.383497 0.383497 0.383497 0.383497 0.385714 0.4 0.414286 0.428571 0.442857 0.457143 0.471429 0.485714 0.5 0.514286 0.528571 0.542857 0.557143 0.571429 0.585714 0.6 0.614286 0.628571 0.642857 0.657143 0.671429 0.685714 0.7 0.714286 0.728571 0.742857 0.757143 0.771429 0.785714 0.8 0.814286 0.828571 0.842857 0.857143 0.871429 0.885714 0.9 0.914286 0.928571 0.942857 0.957143 0.971429 1 1 1 1 1 1
  spline S139 degree 3 poles (8.3445, 178.7545) (8.7365, 178.7362) (9.4313, 178.971) (9.833, 179.5619) (9.9255, 179.8412) knots 0 0 0 0 0.571429 1 1 1 1
  arc A70 (8.3445, 178.7545) -> (6.845, 178.8182) centre (0, 0) ccw
  spline S140 degree 3 poles (5.3618, 180.0351) (5.4303, 179.7489) (5.7805, 179.1261) (6.4529, 178.8332) (6.845, 178.8182) knots 0 0 0 0 0.428571 1 1 1 1
  spline S141 degree 5 poles (5.3618, 180.0351) (5.3601, 180.0423) (5.3472, 180.0963) (5.3229, 180.197) (5.2869, 180.3443) (5.2388, 180.5383) (5.1797, 180.7715) (5.1194, 181.0047) (5.058, 181.2377) (4.9954, 181.4706) (4.9318, 181.7034) (4.867, 181.936) (4.8011, 182.1685) (4.7342, 182.4009) (4.6662, 182.6332) (4.5971, 182.8653) (4.527, 183.0973) (4.4559, 183.3291) (4.3838, 183.5609) (4.3107, 183.7924) (4.2366, 184.0239) (4.1615, 184.2552) (4.0854, 184.4863) (4.0084, 184.7174) (3.9304, 184.9483) (3.8514, 185.179) (3.7716, 185.4096) (3.6908, 185.64) (3.6091, 185.8703) (3.5264, 186.1005) (3.4429, 186.3305) (3.3585, 186.5603) (3.2732, 186.7901) (3.187, 187.0196) (3.1, 187.249) (3.012, 187.4783) (2.9232, 187.7074) (2.8336, 187.9363) (2.7431, 188.1651) (2.6518, 188.3937) (2.5596, 188.6222) (2.4666, 188.8505) (2.3728, 189.0786) (2.2592, 189.3522) (2.1635, 189.58) (2.0864, 189.7621) (2.0281, 189.8986) (1.9891, 189.9896) knots 0.383497 0.383497 0.383497 0.383497 0.383497 0.383497 0.385714 0.4 0.414286 0.428571 0.442857 0.457143 0.471429 0.485714 0.5 0.514286 0.528571 0.542857 0.557143 0.571429 0.585714 0.6 0.614286 0.628571 0.642857 0.657143 0.671429 0.685714 0.7 0.714286 0.728571 0.742857 0.757143 0.771429 0.785714 0.8 0.814286 0.828571 0.842857 0.857143 0.871429 0.885714 0.9 0.914286 0.928571 0.942857 0.957143 0.971429 1 1 1 1 1 1
  arc A71 (1.9891, 189.9896) -> (-1.9891, 189.9896) centre (0, 0) ccw
  spline S142 degree 5 poles (-5.3618, 180.0351) (-5.3601, 180.0423) (-5.3472, 180.0963) (-5.3229, 180.197) (-5.2869, 180.3443) (-5.2388, 180.5383) (-5.1797, 180.7715) (-5.1194, 181.0047) (-5.058, 181.2377) (-4.9954, 181.4706) (-4.9318, 181.7034) (-4.867, 181.936) (-4.8011, 182.1685) (-4.7342, 182.4009) (-4.6662, 182.6332) (-4.5971, 182.8653) (-4.527, 183.0973) (-4.4559, 183.3291) (-4.3838, 183.5609) (-4.3107, 183.7924) (-4.2366, 184.0239) (-4.1615, 184.2552) (-4.0854, 184.4863) (-4.0084, 184.7174) (-3.9304, 184.9483) (-3.8514, 185.179) (-3.7716, 185.4096) (-3.6908, 185.64) (-3.6091, 185.8703) (-3.5264, 186.1005) (-3.4429, 186.3305) (-3.3585, 186.5603) (-3.2732, 186.7901) (-3.187, 187.0196) (-3.1, 187.249) (-3.012, 187.4783) (-2.9232, 187.7074) (-2.8336, 187.9363) (-2.7431, 188.1651) (-2.6518, 188.3937) (-2.5596, 188.6222) (-2.4666, 188.8505) (-2.3728, 189.0786) (-2.2592, 189.3522) (-2.1635, 189.58) (-2.0864, 189.7621) (-2.0281, 189.8986) (-1.9891, 189.9896) knots 0.383497 0.383497 0.383497 0.383497 0.383497 0.383497 0.385714 0.4 0.414286 0.428571 0.442857 0.457143 0.471429 0.485714 0.5 0.514286 0.528571 0.542857 0.557143 0.571429 0.585714 0.6 0.614286 0.628571 0.642857 0.657143 0.671429 0.685714 0.7 0.714286 0.728571 0.742857 0.757143 0.771429 0.785714 0.8 0.814286 0.828571 0.842857 0.857143 0.871429 0.885714 0.9 0.914286 0.928571 0.942857 0.957143 0.971429 1 1 1 1 1 1
  spline S143 degree 3 poles (-6.845, 178.8182) (-6.4529, 178.8332) (-5.7805, 179.1261) (-5.4303, 179.7489) (-5.3618, 180.0351) knots 0 0 0 0 0.571429 1 1 1 1
  arc A72 (-6.845, 178.8182) -> (-8.3445, 178.7545) centre (0, 0) ccw
  spline S144 degree 3 poles (-9.9255, 179.8412) (-9.833, 179.5619) (-9.4313, 178.971) (-8.7365, 178.7362) (-8.3445, 178.7545) knots 0 0 0 0 0.428571 1 1 1 1
  spline S145 degree 5 poles (-9.9255, 179.8412) (-9.9279, 179.8483) (-9.9453, 179.901) (-9.9781, 179.9992) (-10.0264, 180.143) (-10.0908, 180.3322) (-10.1695, 180.5596) (-10.2493, 180.7868) (-10.3303, 181.0137) (-10.4123, 181.2405) (-10.4955, 181.467) (-10.5798, 181.6933) (-10.6651, 181.9194) (-10.7515, 182.1453) (-10.839, 182.3709) (-10.9275, 182.5964) (-11.017, 182.8216) (-11.1075, 183.0466) (-11.199, 183.2713) (-11.2915, 183.4959) (-11.385, 183.7202) (-11.4795, 183.9443) (-11.5749, 184.1682) (-11.6712, 184.3919) (-11.7685, 184.6153) (-11.8667, 184.8385) (-11.9658, 185.0615) (-12.0659, 185.2843) (-12.1668, 185.5068) (-12.2687, 185.7291) (-12.3714, 185.9512) (-12.475, 186.1731) (-12.5795, 186.3947) (-12.6848, 186.6161) (-12.791, 186.8373) (-12.8981, 187.0583) (-13.006, 187.279) (-13.1147, 187.4996) (-13.2243, 187.7198) (-13.3347, 187.9399) (-13.4459, 188.1597) (-13.5579, 188.3793) (-13.6708, 188.5987) (-13.8071, 188.8617) (-13.9218, 189.0805) (-14.0141, 189.2554) (-14.0837, 189.3865) (-14.1303, 189.4738) knots 0.383497 0.383497 0.383497 0.383497 0.383497 0.383497 0.385714 0.4 0.414286 0.428571 0.442857 0.457143 0.471429 0.485714 0.5 0.514286 0.528571 0.542857 0.557143 0.571429 0.585714 0.6 0.614286 0.628571 0.642857 0.657143 0.671429 0.685714 0.7 0.714286 0.728571 0.742857 0.757143 0.771429 0.785714 0.8 0.814286 0.828571 0.842857 0.857143 0.871429 0.885714 0.9 0.914286 0.928571 0.942857 0.957143 0.971429 1 1 1 1 1 1
  arc A73 (-14.1303, 189.4738) -> (-18.0942, 189.1365) centre (0, 0) ccw
  spline S146 degree 5 poles (-20.6105, 178.9318) (-20.6094, 178.9392) (-20.6011, 178.994) (-20.5855, 179.0964) (-20.5622, 179.2463) (-20.5306, 179.4436) (-20.4915, 179.681) (-20.4512, 179.9185) (-20.4098, 180.1558) (-20.3672, 180.3932) (-20.3235, 180.6305) (-20.2787, 180.8678) (-20.2328, 181.1051) (-20.1858, 181.3423) (-20.1378, 181.5795) (-20.0886, 181.8167) (-20.0385, 182.0537) (-19.9873, 182.2908) (-19.9351, 182.5278) (-19.8818, 182.7647) (-19.8276, 183.0016) (-19.7724, 183.2385) (-19.7162, 183.4753) (-19.659, 183.712) (-19.6009, 183.9487) (-19.5418, 184.1853) (-19.4818, 184.4218) (-19.4209, 184.6583) (-19.359, 184.8947) (-19.2962, 185.131) (-19.2325, 185.3673) (-19.1678, 185.6034) (-19.1023, 185.8396) (-19.0359, 186.0756) (-18.9686, 186.3116) (-18.9004, 186.5474) (-18.8314, 186.7832) (-18.7615, 187.019) (-18.6907, 187.2546) (-18.6191, 187.4901) (-18.5466, 187.7256) (-18.4733, 187.961) (-18.3992, 188.1963) (-18.3092, 188.4785) (-18.2332, 188.7136) (-18.1718, 188.9016) (-18.1253, 189.0425) (-18.0942, 189.1365) knots 0.383497 0.383497 0.383497 0.383497 0.383497 0.383497 0.385714 0.4 0.414286 0.428571 0.442857 0.457143 0.471429 0.485714 0.5 0.514286 0.528571 0.542857 0.557143 0.571429 0.585714 0.6 0.614286 0.628571 0.642857 0.657143 0.671429 0.685714 0.7 0.714286 0.728571 0.742857 0.757143 0.771429 0.785714 0.8 0.814286 0.828571 0.842857 0.857143 0.871429 0.885714 0.9 0.914286 0.928571 0.942857 0.957143 0.971429 1 1 1 1 1 1
  spline S147 degree 3 poles (-21.9852, 177.5935) (-21.5958, 177.6418) (-20.9506, 177.9906) (-20.6545, 178.6408) (-20.6105, 178.9318) knots 0 0 0 0 0.571429 1 1 1 1
  arc A74 (-21.9852, 177.5935) -> (-23.4739, 177.4029) centre (0, 0) ccw
  spline S148 degree 3 poles (-25.1414, 178.3516) (-25.0255, 178.0811) (-24.5751, 177.5264) (-23.8629, 177.3514) (-23.4739, 177.4029) knots 0 0 0 0 0.428571 1 1 1 1
  spline S149 degree 5 poles (-25.1414, 178.3516) (-25.1443, 178.3585) (-25.1662, 178.4095) (-25.2071, 178.5046) (-25.2675, 178.6437) (-25.3477, 178.8267) (-25.4454, 179.0467) (-25.5442, 179.2663) (-25.6441, 179.4856) (-25.7451, 179.7045) (-25.8472, 179.9232) (-25.9503, 180.1416) (-26.0546, 180.3596) (-26.1598, 180.5773) (-26.2661, 180.7947) (-26.3734, 181.0119) (-26.4817, 181.2287) (-26.5909, 181.4452) (-26.7012, 181.6614) (-26.8124, 181.8773) (-26.9246, 182.0928) (-27.0377, 182.3081) (-27.1517, 182.5231) (-27.2667, 182.7378) (-27.3826, 182.9522) (-27.4994, 183.1663) (-27.617, 183.38) (-27.7356, 183.5935) (-27.8551, 183.8067) (-27.9754, 184.0196) (-28.0966, 184.2322) (-28.2187, 184.4444) (-28.3416, 184.6564) (-28.4653, 184.8681) (-28.5899, 185.0795) (-28.7153, 185.2906) (-28.8415, 185.5014) (-28.9686, 185.7119) (-29.0964, 185.9221) (-29.2251, 186.132) (-29.3545, 186.3416) (-29.4848, 186.5509) (-29.6158, 186.7599) (-29.774, 187.0104) (-29.9068, 187.2187) (-30.0136, 187.3852) (-30.0941, 187.5098) (-30.1479, 187.5929) knots 0.383497 0.383497 0.383497 0.383497 0.383497 0.383497 0.385714 0.4 0.414286 0.428571 0.442857 0.457143 0.471429 0.485714 0.5 0.514286 0.528571 0.542857 0.557143 0.571429 0.585714 0.6 0.614286 0.628571 0.642857 0.657143 0.671429 0.685714 0.7 0.714286 0.728571 0.742857 0.757143 0.771429 0.785714 0.8 0.814286 0.828571 0.842857 0.857143 0.871429 0.885714 0.9 0.914286 0.928571 0.942857 0.957143 0.971429 1 1 1 1 1 1
  arc A75 (-30.1479, 187.5929) -> (-34.0689, 186.9206) centre (0, 0) ccw